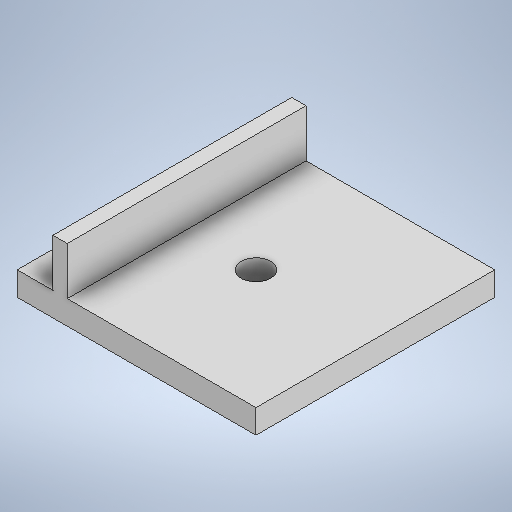
# Autodesk Inventor part: horony_upper
Saved by Autodesk Inventor 2025.2 (Build 292293000, 293)
## iProperties
Created: 2025-08-23
Part Number: horony_upper
Material: Generic
Document SubType Name: Modeling
Designer: MB
Density: 1 g/cm^3
Appearance: Default
Author: MB
Autodesk Inventor part; units mm, degrees
ref_plane "YZ Plane" through (0, 0, 0) normal (1, 0, 0) x (0, 1, 0)
ref_plane "XZ Plane" through (0, 0, 0) normal (0, 1, 0) x (-1, 0, 0)
ref_plane "XY Plane" through (0, 0, 0) normal (0, 0, 1) x (1, 0, 0)
sketch "Sketch1" plane through (0, 0, 0) normal (0, 1, 0) x (-1, 0, 0)
  line L0 (0, 0) -> (-50, 0)
  line L1 (-50, 0) -> (-50, 50)
  line L2 (-50, 50) -> (0, 50)
  line L3 (0, 50) -> (0, 0)
  dimension "d0" = 50
  dimension "d1" = 50
  constraints: 8 end point, 2 parallel, 1 horizontal, 1 perpendicular
  measures "d0" distance of L1.end L2.end
  measures "d1" distance of L0.end L1.end
extrude "Extrusion1" add sketch "Sketch1" along normal blind 5
sketch "Sketch2" plane through (0, 5, 0) normal (0, 1, 0) x (1, 0, 0)
  line L0 (0, -50) -> (50, -50) projected
  line L1 (0, 0) -> (0, -50) projected
  point P0 (25, -25)
  dimension "d4" = 25
  dimension "d12" = 25
  measures "d4" distance from line of L0 point (25, -25)
  measures "d12" distance from line of L1 point (25, -25)
hole "Hole1" at (25, 5, 25) direction (0, -1, 0) diameter 6.2 end through all
sketch "Sketch3" plane through (0, 5, 0) normal (0, 1, 0) x (1, 0, 0)
  line L0 (50, 0) -> (0, 0) projected
  line L1 (0, -50) -> (50, -50) projected
  line L2 (7.4764, 0) -> (10.4764, 0)
  line L3 (10.4764, 0) -> (10.4764, -50)
  line L4 (10.4764, -50) -> (7.4764, -50)
  line L5 (7.4764, -50) -> (7.4764, 0)
  dimension "d13" = 3
  constraints: 8 end point, 2 parallel, 2 point on line, 1 horizontal, 1 perpendicular
  measures "d13" distance of L3.end L4.end
extrude "Extrusion2" add sketch "Sketch3" along normal blind 10
body "Solid1"
